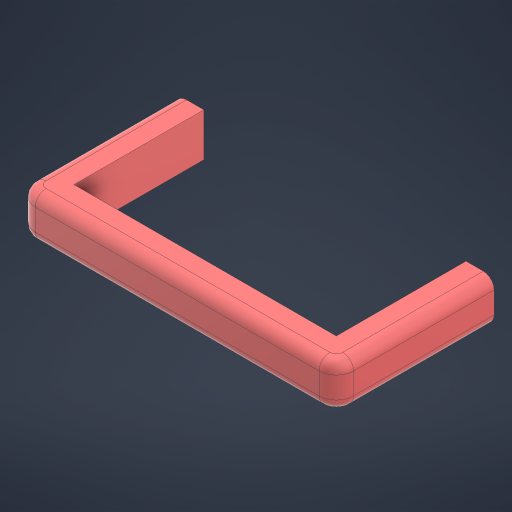
# Autodesk Inventor part: Bumpers
Saved by Autodesk Inventor 2024.3 (Build 283343000, 343)
## iProperties
Created: 2024-11-27
Part Number: Bumpers
Material: Generic
Document SubType Name: Modeling
Designer: kaito
Density: 1 g/cm^3
Appearance: Default
Author: kaito
Autodesk Inventor part; units mm, degrees
ref_plane "YZ Plane" through (0, 0, 0) normal (1, 0, 0) x (0, 1, 0)
ref_plane "XZ Plane" through (0, 0, 0) normal (0, 1, 0) x (-1, 0, 0)
ref_plane "XY Plane" through (0, 0, 0) normal (0, 0, 1) x (1, 0, 0)
sketch "Sketch1" plane through (0, 0, 0) normal (0, 1, 0) x (-1, 0, 0)
  line L0 (0, 0) -> (808.3618, 0)
  line L1 (808.3618, 0) -> (808.3618, -19.05)
  line L2 (808.3618, -19.05) -> (0, -19.05)
  line L3 (0, -19.05) -> (0, 0)
  line L4 (0, -19.05) -> (19.05, -19.05)
  line L5 (19.05, -19.05) -> (19.05, -400.05)
  line L6 (19.05, -400.05) -> (0, -400.05)
  line L7 (0, -400.05) -> (0, -19.05)
  line L8 (808.3618, -19.05) -> (789.3118, -19.05)
  line L9 (789.3118, -19.05) -> (789.3118, -400.05)
  line L10 (789.3118, -400.05) -> (808.3618, -400.05)
  line L11 (808.3618, -400.05) -> (808.3618, -19.05)
  point P0 (789.3118, -19.05)
  dimension "d0" = 808.3618
  dimension "d1" = 19.05
  dimension "d2" = 381
  dimension "d3" = 19.05
  constraints: 24 end point, 6 parallel, 3 horizontal, 3 perpendicular, 2 equal length
  measures "d0" distance of L1.end L2.end
  measures "d1" distance of L0.end L1.end
  measures "d2" distance of L4.end L5.end
  measures "d3" distance of L5.end L6.end
extrude "Extrusion1" add sketch "Sketch1" along normal blind 127
sketch "Sketch2" plane through (0, 0, -400.05) normal (0, 0, -1) x (-1, 0, 0)
  circle A0 centre (-31.75, 95.25) radius 31.75
  line L0 (0, 0) -> (0, 127) projected
  circle A1 centre (-31.75, 31.75) radius 31.75
  line L1 (-62.6379, 0) -> (0, 0)
  line L2 (808.3618, 127) -> (0, 127) projected
  line L3 (0, 127) -> (-31.75, 127)
  line L4 (-63.5, 95.25) -> (-63.5, 31.75)
  point P0 (-31.75, 0)
  dimension "d7" = 63.5
  dimension "d6" = 63.5
  constraints: 6 end point, 2 horizontal, 2 point on circle, 2 tangent, 1 centre point, 1 collinear, 1 perpendicular, 1 vertical, 4 other
  measures "d6" diameter of A0
sketch3d "3D Sketch1"
  line L0 (0, 127, -400.05) -> (0, 127, 0)
  line L1 (0, 127, 0) -> (-808.3618, 127, 0)
  line L2 (-808.3618, 127, 0) -> (-808.3618, 127, -400.05)
sweep "Sweep1" add profiles "Sketch2" path "3D Sketch1"
fillet "Fillet1" radius 50.8 3 edges at (54.2006, 117.7006, 54.2006) (54.2006, 9.2994, 54.2006) (63.5, 63.5, 63.5)
fillet "Fillet2" radius 50.8 3 edges at (-862.5624, 117.7006, 54.2006) (-862.5624, 9.2994, 54.2006) (-871.8618, 63.5, 63.5)
body "Solid1"
